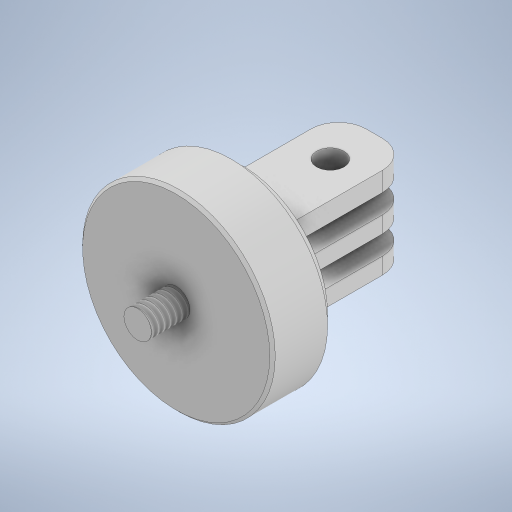
# Autodesk Inventor part: Go Pro Mount with threaded mount
Saved by Autodesk Inventor 2023.5 (Build 275446000, 446)
## iProperties
Created: 2024-07-11
Part Number: Go Pro Mount with threaded mount
Material: Generic
Document SubType Name: Modeling
Designer: Big Sean T
Density: 1 g/cm^3
Appearance: Default
Author: Big Sean T
Autodesk Inventor part; units mm, degrees
ref_plane "YZ Plane" through (0, 0, 0) normal (1, 0, 0) x (0, 1, 0)
ref_plane "XZ Plane" through (0, 0, 0) normal (0, 1, 0) x (-1, 0, 0)
ref_plane "XY Plane" through (0, 0, 0) normal (0, 0, 1) x (1, 0, 0)
sketch "Sketch1" plane through (0, 0, 0) normal (0, 0, 1) x (1, 0, 0)
  line L0 (0, 0) -> (17.5, 0)
  circle A0 centre (17.5, 0) radius 17.5
  dimension "d0" = 17.5
  constraints: 2 end point, 1 coincident, 1 horizontal, 1 horizontal alignment, 2 other
  measures "d0" distance of L0.start L0.end
extrude "Extrusion1" add sketch "Sketch1" along normal blind 12
chamfer "Chamfer1" distance 0.5 angle 45 1 edges at (0, 0, 12)
chamfer "Chamfer2" distance 2 angle 45 1 edges at (0, 0, 0)
sketch "Sketch5" plane through (17.5, 0, 0) normal (0, 0, -1) x (-1, 0, 0)
  line L0 (6.5, 1.5) -> (-6.5, 1.5)
  line L1 (-6.5, 1.5) -> (-6.5, -1.5)
  line L2 (-6.5, -1.5) -> (6.5, -1.5)
  line L3 (6.5, -1.5) -> (6.5, 1.5)
  line L4 (6.5, 1.5) -> (-6.5, -1.5) construction
  line L5 (-6.5, 1.5) -> (6.5, -1.5) construction
  point P0 (17.5, 0)
  point P1 (0, 0)
  dimension "d21" = 3
  dimension "d22" = 13
  constraints: 12 end point, 2 midpoint, 2 parallel, 1 horizontal, 1 perpendicular
  measures "d21" distance of L0.end L1.end
  measures "d22" distance of L1.end L2.end
extrude "Extrusion3" add sketch "Sketch5" along normal blind 24
sketch "Sketch6" plane through (17.5, 0, 0) normal (0, 0, -1) x (-1, 0, 0)
  line L0 (-6.5, -1.5) -> (6.5, -1.5) projected
  line L1 (0, -1.5) -> (0, -5)
  line L2 (0, -5) -> (-6.5, -5)
  line L3 (-6.5, -5) -> (-6.5, -8)
  line L4 (-6.5, -8) -> (6.5, -8)
  line L5 (6.5, -8) -> (6.5, -5)
  line L6 (6.5, -5) -> (0, -5)
  point P0 (17.5, 0)
  dimension "d25" = 3.5
  dimension "d26" = 3
  constraints: 12 end point, 3 perpendicular, 2 horizontal, 2 midpoint, 1 point on line, 1 vertical
  measures "d25" distance of point (0, -1.5) L1.end
  measures "d26" distance of L2.end L3.end
extrude "Extrusion4" add sketch "Sketch6" along normal blind 24
sketch "Sketch7" plane through (17.5, 0, 0) normal (0, 0, -1) x (-1, 0, 0)
  line L0 (-6.5, 1.5) -> (6.5, 1.5) projected
  line L1 (0, 1.5) -> (0, 5)
  line L2 (0, 5) -> (6.5, 5)
  line L3 (6.5, 5) -> (6.5, 8.5)
  line L4 (6.5, 8.5) -> (-6.5, 8.5)
  line L5 (-6.5, 8.5) -> (-6.5, 5)
  line L6 (-6.5, 5) -> (0, 5)
  point P0 (17.5, 0)
  dimension "d29" = 3.5
  dimension "d30" = 3.5
  constraints: 12 end point, 2 horizontal, 2 perpendicular, 1 collinear, 1 midpoint, 1 point on line, 1 vertical
  measures "d29" distance of L1.start L1.end
  measures "d30" distance of L2.end L3.end
extrude "Extrusion5" add sketch "Sketch7" along normal blind 24
fillet "Fillet1" radius 5 1 edges at (24, -6.5, -24)
fillet "Fillet2" radius 5 1 edges at (11, -6.5, -24)
fillet "Fillet3" radius 5 1 edges at (24, 0, -24)
fillet "Fillet4" radius 5 1 edges at (11, 0, -24)
fillet "Fillet5" radius 5 1 edges at (24, 6.75, -24)
fillet "Fillet6" radius 5 1 edges at (11, 6.75, -24)
sketch "Sketch8" plane through (11, -8, 0) normal (0, -1, 0) x (1, 0, 0)
  line L0 (5, -24) -> (8, -24) projected
  circle A0 centre (6.5, -16) radius 2.5
  point P0 (-11, 0)
  constraints: 1 centre point
extrude "Extrusion6" cut sketch "Sketch8" against normal blind 24
fillet "Face Fillet1" radius 1.5 1 edges at (17.5, -8, 0)
fillet "Face Fillet2" radius 1.4986 1 edges at (17.5, -5, 0)
fillet "Face Fillet3" radius 1.4986 1 edges at (17.5, -1.5, 0)
fillet "Face Fillet4" radius 1.4986 1 edges at (17.5, 1.5, 0)
fillet "Face Fillet5" radius 1.4986 1 edges at (17.5, 5, 0)
fillet "Face Fillet6" radius 1.4986 1 edges at (17.5, 8.5, 0)
fillet "Face Fillet7" radius 1.4986 3 edges at (11, 9.2493, 0) (11, 6.75, 0) (11, 4.2507, 0)
fillet "Face Fillet8" radius 1.4986 3 edges at (11, 2.2493, 0) (11, 0, 0) (11, -2.2493, 0)
fillet "Face Fillet9" radius 1.4986 3 edges at (11, -4.2507, 0) (11, -6.5, 0) (11, -8.75, 0)
fillet "Face Fillet10" radius 1.4986 3 edges at (24, -8.75, 0) (24, -6.5, 0) (24, -4.2507, 0)
fillet "Face Fillet11" radius 1.4986 3 edges at (24, -2.2493, 0) (24, 0, 0) (24, 2.2493, 0)
fillet "Face Fillet12" radius 1.4986 3 edges at (24, 4.2507, 0) (24, 6.75, 0) (24, 9.2493, 0)
sketch "Sketch11" plane through (17.5, 0, 12) normal (0, 0, 1) x (1, 0, 0)
  circle A0 centre (0, 0) radius 2.5
  point P0 (-17.5, 0)
  dimension "d60" = 5
  constraints: 1 centre point
  measures "d60" diameter of A0
extrude "Extrusion8" add sketch "Sketch11" along normal blind 7
thread "Thread3" size "12-24 UNC" class "2A" standard "ANSI Unified Screw Threads" full length
body "Solid1"
